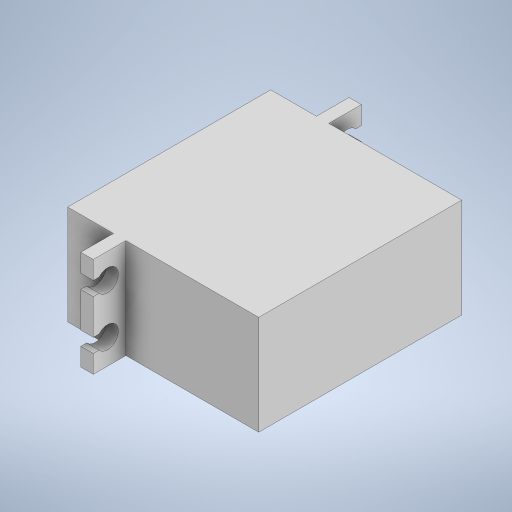
# Autodesk Inventor part: MG996R
Saved by Autodesk Inventor 2024 (Build 280153000, 153)
## iProperties
Created: 2024-04-17
Part Number: MG996R
Material: Generic
Document SubType Name: Modeling
Designer: compu
Density: 1 g/cm^3
Appearance: Default
Author: compu
Autodesk Inventor part; units mm, degrees
ref_plane "YZ Plane" through (0, 0, 0) normal (1, 0, 0) x (0, 1, 0)
ref_plane "XZ Plane" through (0, 0, 0) normal (0, 1, 0) x (-1, 0, 0)
sketch "Sketch1" plane through (0, 0, 0) normal (1, 0, 0) x (0, 1, 0)
  line L0 (20, 20.4) -> (0, 20.4)
  line L1 (0, 20.4) -> (0, -20.4)
  line L2 (0, -20.4) -> (20, -20.4)
  line L3 (20, -20.4) -> (20, 20.4)
  line L4 (0, -28.56) -> (0, 28.56) projected
  line L5 (-4, 0) -> (24, 0) projected
  point P0 (0, 0)
  dimension "d0" = 40.8
  dimension "d1" = 20
  constraints: 8 end point, 2 parallel, 1 collinear, 1 horizontal, 1 perpendicular, 1 other
  measures "d0" distance of L0.end L1.end
  measures "d1" distance of L1.end L2.end
extrude "Extrusion1" add sketch "Sketch1" along normal blind 38.4
sketch "Sketch2" plane through (0, 0, 0) normal (1, 0, 0) x (0, 1, 0)
  line L0 (20, 20.4) -> (0, 20.4) projected
  line L1 (20, -20.4) -> (20, 20.4) projected
  line L2 (0, -20.4) -> (20, -20.4) projected
  line L3 (0, 20.4) -> (0, -20.4) projected
  line L4 (10, 20.4) -> (10, -20.4)
  line L5 (0, 20.4) -> (0, -20.4) projected
  circle A0 centre (10, 10.35) radius 2.95
  point P0 (0, 0)
  dimension "d4" = 5.9
  dimension "d40" = 10.05
  constraints: 2 end point, 2 midpoint, 1 centre point, 1 parallel, 1 point on line
  measures "d4" diameter of A0
  measures "d40" distance from line of L0 A0.centre
extrude "Extrusion2" add sketch "Sketch2" against normal blind 3.5 contours A0 L4 | L4 A0
sketch "Sketch3" plane through (0, 0, 20.4) normal (0, 0, 1) x (1, 0, 0)
  line L0 (9.2, 20) -> (11.7, 20)
  line L1 (11.7, 20) -> (11.7, 0)
  line L2 (11.7, 0) -> (9.2, 0)
  line L3 (9.2, 0) -> (9.2, 20)
  line L4 (0, 20) -> (0, 0) projected
  line L5 (0, 0) -> (38.4, 0) projected
  line L6 (38.4, 20) -> (38.4, 0) projected
  line L7 (0, 20) -> (38.4, 20) projected
  point P0 (0, 0)
  dimension "d7" = 2.5
  dimension "d9" = 9.2
  dimension "d10" = 26.7
  constraints: 8 end point, 2 collinear, 2 parallel, 1 horizontal, 1 perpendicular
  measures "d7" distance of L1.end L2.end
  measures "d9" distance between parallel lines of L4 L3
  measures "d10" distance between parallel lines of L6 L1
extrude "Extrusion3" add sketch "Sketch3" along normal blind 6.55 contours L0 L1 L2 L3
sketch "Sketch4" plane through (0, 0, -20.4) normal (0, 0, -1) x (-1, 0, 0)
  line L0 (-11.7, 20) -> (-9.2, 20)
  line L1 (-9.2, 20) -> (-9.2, 0)
  line L2 (-9.2, 0) -> (-11.7, 0)
  line L3 (-11.7, 0) -> (-11.7, 20)
  line L4 (0, 0) -> (0, 20) projected
  line L5 (0, 20) -> (-38.4, 20) projected
  line L6 (-38.4, 0) -> (-38.4, 20) projected
  line L7 (0, 0) -> (-38.4, 0) projected
  point P0 (0, 0)
  dimension "d13" = 2.5
  dimension "d14" = 9.2
  dimension "d15" = 26.7
  constraints: 8 end point, 2 collinear, 2 parallel, 1 horizontal, 1 perpendicular
  measures "d13" distance of L1.end L2.end
  measures "d14" distance between parallel lines of L4 L1
  measures "d15" distance between parallel lines of L6 L3
extrude "Extrusion4" add sketch "Sketch4" along normal blind 6.55 contours L0 L1 L2 L3
sketch "Sketch5" plane through (9.2, 0, 20.4) normal (-1, 0, 0) x (0, 0, 1)
  circle A0 centre (-10.05, 10) radius 2.95 projected
  line L0 (0, 20) -> (0, 0) projected
  line L1 (-40.8, 20) -> (0, 20) projected
  line L2 (-40.8, 0) -> (-40.8, 20) projected
  line L3 (0, 0) -> (-40.8, 0) projected
  line L4 (0, 20) -> (0, 0) projected
  line L5 (0, 20) -> (6.55, 20) projected
  line L6 (6.55, 0) -> (6.55, 20) projected
  line L7 (0, 0) -> (6.55, 0) projected
  line L8 (-40.8, 0) -> (-40.8, 20) projected
  line L9 (-40.8, 0) -> (-47.35, 0) projected
  line L10 (-47.35, 20) -> (-47.35, 0) projected
  line L11 (-40.8, 20) -> (-47.35, 20) projected
  circle A1 centre (3.7, 14.95) radius 2.2
  arc A2 (5.3971, 6.45) -> (5.3971, 3.65) centre (3.7, 5.05) ccw
  circle A3 centre (-44.5, 14.95) radius 2.2
  circle A4 centre (-44.5, 5.05) radius 2.2
  line L12 (-47.35, 10) -> (6.55, 10) construction
  line L13 (-20.4, 0) -> (-20.4, 20) construction
  line L14 (6.55, 6.45) -> (5.3971, 6.45)
  line L15 (5.3971, 3.65) -> (6.55, 3.65)
  line L16 (6.55, 3.65) -> (6.55, 6.45)
  line L17 (3.7, 5.05) -> (6.55, 5.05) construction
  line L18 (3.7, 5.05) -> (3.7, 20) construction
  line L19 (-44.5, 5.05) -> (6.55, 5.05) construction
  point P0 (6.55, 3.65)
  point P1 (6.55, 6.45)
  dimension "d18" = 4.4
  dimension "d19" = 4.4
  dimension "d20" = 4.4
  dimension "d21" = 4.4
  dimension "d22" = 48.2
  dimension "d23" = 48.2
  dimension "d24" = 9.9
  dimension "d25" = 9.9
  dimension "d26" = 24.1
  dimension "d27" = 4.95
  dimension "d28" = 2.8
  constraints: 16 end point, 4 centre point, 4 midpoint, 3 point on line, 2 point on circle, 1 collinear, 1 horizontal, 1 parallel, 1 perpendicular, 1 other
  measures "d18" diameter of A1
  measures "d19" diameter of A2
  measures "d20" diameter of A3
  measures "d21" diameter of A4
  measures "d22" distance of L19.start L17.start
  measures "d23" distance of A3.centre A1.centre
  measures "d24" distance of L17.start A1.centre
  measures "d25" distance of L19.start A3.centre
  measures "d26" distance from line of L13 L19.start
  measures "d27" distance from line of L12 L19.start
  measures "d28" distance between parallel lines of L15 L14
extrude "Extrusion5" cut sketch "Sketch5" against normal blind 6.55 contours L6 L15 A2 L14 | A1 | A3 | A4
ref_plane "Work Plane1" through (9.2, 14.95, 24.1) normal (0, 0, -1) x (1, 0, 0)
sketch "Sketch6" plane through (9.2, 14.95, 24.1) normal (0, 0, -1) x (1, 0, 0)
  line L0 (2.5, 2.2) -> (2.5, -2.2) projected
  line L1 (0, -2.2) -> (0, 2.2) projected
  line L2 (-21.08, 0) -> (37.58, 0) projected
  line L3 (0, -2.2) -> (2.5, -2.2) projected
  line L4 (0, 2.2) -> (2.5, 2.2) projected
  line L5 (0, 1.4) -> (2.5, 1.4)
  line L6 (2.5, 1.4) -> (2.5, -1.4)
  line L7 (2.5, -1.4) -> (0, -1.4)
  line L8 (0, -1.4) -> (0, 1.4)
  point P0 (-9.2, 14.95)
  point P1 (0, -1.4)
  point P2 (2.5, -1.4)
  point P3 (2.5, 1.4)
  point P4 (0, 1.4)
  dimension "d31" = 2.8
  constraints: 8 end point, 2 collinear, 2 parallel, 1 horizontal, 1 perpendicular, 1 other
  measures "d31" distance between parallel lines of L5 L7
extrude "Extrusion6" cut sketch "Sketch6" against normal blind 6.55 contours L0 L2 L1 L5 | L0 L7 L1 L2
sketch "Sketch7" plane through (0, 0, -26.95) normal (0, 0, -1) x (-1, 0, 0)
  line L0 (-12.71, 16.35) -> (-7.7221, 16.35)
  line L1 (-7.7221, 16.35) -> (-7.7221, 13.55)
  line L2 (-7.7221, 13.55) -> (-12.71, 13.55)
  line L3 (-12.71, 13.55) -> (-12.71, 16.35)
  line L4 (-13.2403, 6.45) -> (-6.6781, 6.45)
  line L5 (-6.6781, 6.45) -> (-6.6781, 3.65)
  line L6 (-6.6781, 3.65) -> (-13.2403, 3.65)
  line L7 (-13.2403, 3.65) -> (-13.2403, 6.45)
  line L8 (11.88, 14.95) -> (-46.78, 14.95) projected
  line L9 (11.88, 5.05) -> (-46.78, 5.05) projected
  point P0 (0, 0)
  dimension "d34" = 2.8
  dimension "d35" = 2.8
  constraints: 16 end point, 4 parallel, 2 horizontal, 2 perpendicular, 2 other
  measures "d34" distance of L0.end L1.end
  measures "d35" distance of L4.end L5.end
extrude "Extrusion7" cut sketch "Sketch7" against normal up to surface contours L0 L1 L8 L3 | L8 L1 L2 L3
extrude "Extrusion8" cut sketch "Sketch7" against normal up to surface contours L4 L5 L9 L7 | L9 L5 L6 L7
body "Solid1"
